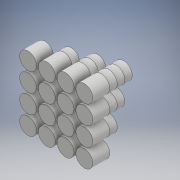
# Autodesk Inventor part: 圓柱
Saved by Autodesk Inventor 2017 (Build 210142000, 142)
## iProperties
Created: 2021-05-20
Part Number: 圓柱
Material: Generic
Document SubType Name: Modeling
Designer: user
Density: 1 g/cm^3
Appearance: Default
Author: user
Autodesk Inventor part; units mm, degrees
ref_plane "YZ Plane" through (0, 0, 0) normal (1, 0, 0) x (0, 1, 0)
ref_plane "XZ Plane" through (0, 0, 0) normal (0, 1, 0) x (-1, 0, 0)
ref_plane "XY Plane" through (0, 0, 0) normal (0, 0, 1) x (1, 0, 0)
sketch "Sketch1" plane through (0, 0, 0) normal (0, 1, 0) x (-1, 0, 0)
  circle A0 centre (0, 0) radius 45
  dimension "d0" = 90
  constraints: 1 centre point, 1 coincident
  measures "d0" diameter of A0
extrude "Extrusion1" add sketch "Sketch1" along normal blind 90
pattern_linear "Rectangular Pattern1" count 4 spacing 100 along (1, 0, 0) count 4 spacing 100 along (0, 0, 1)
sketch "Sketch2" plane through (0, 90, 0) normal (0, 1, 0) x (1, 0, 0)
  circle A0 centre (100, -100) radius 45 projected
  line L0 (0, 0) -> (100, -100)
  circle A1 centre (50, -50) radius 45
  dimension "d9" = 90
  constraints: 2 end point, 1 centre point, 1 midpoint
  measures "d9" diameter of A1
extrude "Extrusion2" add sketch "Sketch2" along normal blind 90 separate body contours A1 L0 A0 | A0 L0 A1 | A1 L0 A0 | A0 L0 A1
pattern_linear "Rectangular Pattern2" count 3 spacing 100 along (1, 0, 0) count 3 spacing 100 along (0, 0, 1) bodies 2
sketch "Sketch3" plane through (50, 180, 150) normal (0, 1, 0) x (1, 0, 0)
  circle A0 centre (50, 50) radius 45 projected
  point P0 (-50, 150)
extrude "Extrusion3" add sketch "Sketch3" along normal blind 90 separate body
pattern_linear "Rectangular Pattern3" count 2 spacing 100 along (1, 0, 0) count 2 spacing 100 along (0, 0, 1) bodies 3
sketch "Sketch4" plane through (100, 270, 200) normal (0, 1, 0) x (1, 0, 0)
  circle A0 centre (50, 50) radius 45 projected
  point P0 (-100, 200)
extrude "Extrusion4" add sketch "Sketch4" along normal blind 90 separate body
body "Solid1"
body "Solid2"
body "Solid3"
body "Solid4"
body "Solid5"
body "Solid6"
body "Solid7"
body "Solid8"
body "Solid9"
body "Solid10"
body "Solid11"
body "Solid12"
body "Solid13"
body "Solid14"
body "Solid15"
body "Solid16"
body "Solid17"
body "Solid18"
body "Solid19"
body "Solid20"
body "Solid21"
body "Solid22"
body "Solid23"
body "Solid24"
body "Solid25"
body "Solid26"
body "Solid27"
body "Solid28"
body "Solid29"
body "Solid30"
